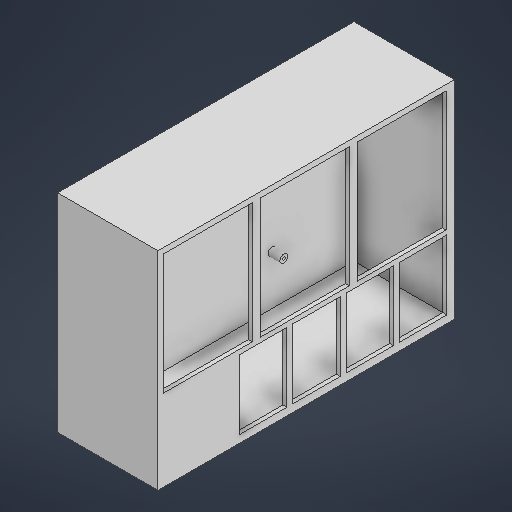
# Autodesk Inventor part: Part1
Saved by Autodesk Inventor 2026 (Build 300175000, 175)
## iProperties
Created: 2025-05-11
Part Number: Part1
Material: Generic
Document SubType Name: Modeling
Designer: Riley
Density: 1 g/cm^3
Appearance: Default
Author: Riley
Autodesk Inventor part; units mm, degrees
ref_plane "YZ Plane" through (0, 0, 0) normal (1, 0, 0) x (0, 1, 0)
ref_plane "XZ Plane" through (0, 0, 0) normal (0, 1, 0) x (-1, 0, 0)
ref_plane "XY Plane" through (0, 0, 0) normal (0, 0, 1) x (1, 0, 0)
sketch "Sketch1" plane through (0, 0, 0) normal (1, 0, 0) x (0, 1, 0)
  line L0 (0, 0) -> (-210, 0)
  line L1 (-210, 0) -> (-210, -300)
  line L2 (-210, -300) -> (0, -300)
  line L3 (0, -300) -> (0, 0)
  dimension "d0" = 210
  dimension "d1" = 300
  constraints: 8 end point, 2 parallel, 1 horizontal, 1 perpendicular
  measures "d0" distance of L2.end L1.end
  measures "d1" distance of L1.end L0.end
extrude "Extrusion1" add sketch "Sketch1" along normal blind 101.6
sketch "Sketch2" plane through (101.6, 0, 0) normal (1, 0, 0) x (0, 0, -1)
  line L0 (0, -210) -> (300, -210) projected
  line L1 (300, -210) -> (300, 0) projected
  line L2 (300, 0) -> (0, 0) projected
  line L3 (0, 0) -> (0, -210) projected
  line L4 (1.6, -1.6) -> (298.4, -1.6)
  line L5 (298.4, -1.6) -> (298.4, -208.4)
  line L6 (298.4, -208.4) -> (1.6, -208.4)
  line L7 (1.6, -208.4) -> (1.6, -1.6)
  dimension "d4" = 1.6
  constraints: 8 end point, 3 other
  measures "d4" distance between parallel lines of L2 L4
extrude "Extrusion2" cut sketch "Sketch2" against normal blind 100 contours L4 L5 L6 L7
sketch "Sketch3" plane through (1.6, 0, 0) normal (1, 0, 0) x (0, 0, -1)
  circle A0 centre (75.3333, -47.4667) radius 4
  circle A1 centre (215.3333, -47.4667) radius 4
  circle A2 centre (215.3333, -158.4667) radius 4
  circle A3 centre (75.3333, -158.4667) radius 4
  point P0 (0, 0)
  dimension "d7" = 8
  dimension "d8" = 8
  dimension "d9" = 8
  dimension "d10" = 8
  dimension "d11" = 140
  dimension "d12" = 111
  constraints: 4 centre point, 2 horizontal alignment, 2 vertical alignment
  measures "d7" diameter of A0
  measures "d8" diameter of A1
  measures "d9" diameter of A2
  measures "d10" diameter of A3
  measures "d11" distance of A1.centre A0.centre
  measures "d12" distance of A2.centre A1.centre
extrude "Extrusion3" add sketch "Sketch3" along normal blind 12
sketch "Sketch4" plane through (13.6, -47.4667, -75.3333) normal (1, 0, 0) x (0, 0, -1)
  circle A0 centre (0, 0) radius 4 projected
  circle A1 centre (140, 0) radius 4 projected
  circle A2 centre (140, -111) radius 4 projected
  circle A3 centre (0, -111) radius 4 projected
  point P0 (-75.3333, 47.4667)
hole "Hole1" at (13.6, -47.4667, -75.3333) at (13.6, -47.4667, -215.3333) at (13.6, -158.4667, -215.3333) at (13.6, -158.4667, -75.3333) direction (-1, 0, 0) diameter 2.8 depth 10.4
sketch "Sketch5" plane through (101.6, 0, 0) normal (1, 0, 0) x (0, 0, -1)
  line L0 (5.6, -5.6) -> (95.6, -5.6)
  line L1 (95.6, -5.6) -> (95.6, -127.6)
  line L2 (95.6, -127.6) -> (5.6, -127.6)
  line L3 (5.6, -127.6) -> (5.6, -5.6)
  line L4 (1.6, -208.4) -> (1.6, -1.6) projected
  line L5 (1.6, -1.6) -> (298.4, -1.6) projected
  line L6 (103.6, -5.6) -> (193.6, -5.6)
  line L7 (103.6, -127.6) -> (103.6, -5.6)
  line L8 (193.6, -5.6) -> (193.6, -127.6)
  line L9 (193.6, -127.6) -> (103.6, -127.6)
  line L10 (201.6, -5.6) -> (291.6, -5.6)
  line L11 (201.6, -127.6) -> (201.6, -5.6)
  line L12 (291.6, -5.6) -> (291.6, -127.6)
  line L13 (291.6, -127.6) -> (201.6, -127.6)
  line L14 (298.4, -1.6) -> (298.4, -208.4) projected
  line L15 (292.4, -132.4) -> (244.4, -132.4)
  line L16 (244.4, -132.4) -> (244.4, -202.4)
  line L17 (244.4, -202.4) -> (292.4, -202.4)
  line L18 (292.4, -202.4) -> (292.4, -132.4)
  line L19 (298.4, -208.4) -> (1.6, -208.4) projected
  line L20 (190.4, -132.4) -> (190.4, -202.4)
  line L21 (238.4, -132.4) -> (190.4, -132.4)
  line L22 (238.4, -202.4) -> (238.4, -132.4)
  line L23 (190.4, -202.4) -> (238.4, -202.4)
  line L24 (136.4, -132.4) -> (136.4, -202.4)
  line L25 (184.4, -132.4) -> (136.4, -132.4)
  line L26 (184.4, -202.4) -> (184.4, -132.4)
  line L27 (136.4, -202.4) -> (184.4, -202.4)
  line L28 (82.4, -132.4) -> (82.4, -202.4)
  line L29 (130.4, -132.4) -> (82.4, -132.4)
  line L30 (130.4, -202.4) -> (130.4, -132.4)
  line L31 (82.4, -202.4) -> (130.4, -202.4)
  point P0 (0, 0)
  point P1 (268.4, -202.4)
  point P2 (214.4, -202.4)
  point P3 (160.4, -202.4)
  point P4 (106.4, -202.4)
  dimension "d22" = 90
  dimension "d23" = 122
  dimension "d24" = 4
  dimension "d25" = 4
  dimension "d28" = 98
  dimension "d33" = 6.8
  dimension "d34" = 48
  dimension "d35" = 70
  dimension "d36" = 6
  dimension "d37" = 6
  dimension "d40" = 54
  constraints: 56 end point, 4 horizontal, 4 parallel, 2 perpendicular, 1 collinear, 1 midpoint, 42 other
  measures "d22" distance between parallel lines of L3 L1
  measures "d23" distance between parallel lines of L2 L0
  measures "d24" distance between parallel lines of L4 L3
  measures "d25" distance between parallel lines of L5 L0
  measures "d28" distance of L0.start L6.start
  measures "d33" distance between parallel lines of L14 L12
  measures "d34" distance between parallel lines of L18 L16
  measures "d35" distance from line of point (268.4, -202.4) L15
  measures "d36" distance between parallel lines of L14 L18
  measures "d37" distance between parallel lines of L19 L17
  measures "d40" distance of L15.end L20.start
extrude "Extrusion4" add sketch "Sketch5" against normal blind 4
equation "\"d8\" = d7"
equation "\"d9\" = d7"
equation "\"d10\" = d7"
equation "\"d25\" = d24"
equation "\"d37\" = d36"
body "Solid1"
